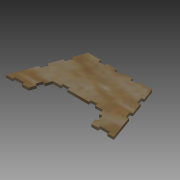
# Autodesk Inventor part: back
Saved by Autodesk Inventor 2016 (Build 200138000, 138)
## iProperties
Created: 2015-10-06
Part Number: back
Material: Generic
Document SubType Name: Modeling
Designer: Haukur
Density: 1 g/cm^3
Appearance: Plywood - Weathered
Author: Haukur
Autodesk Inventor part; units mm, degrees
ref_plane "YZ Plane" through (0, 0, 0) normal (1, 0, 0) x (0, 1, 0)
ref_plane "XZ Plane" through (0, 0, 0) normal (0, 1, 0) x (-1, 0, 0)
ref_plane "XY Plane" through (0, 0, 0) normal (0, 0, 1) x (1, 0, 0)
sketch "Sketch1" plane through (0, 0, 0) normal (0, 0, 1) x (1, 0, 0)
  line L0 (-6.8404, -18.7939) -> (73.1596, -18.7939) construction
  line L1 (126.5636, -18.7939) -> (116.303, 9.3969)
  line L2 (27.3616, 75.1754) -> (20.5212, 56.3816)
  line L3 (20.5212, 56.3816) -> (24.28, 55.0135)
  line L4 (24.28, 55.0135) -> (20.8598, 45.6166)
  line L5 (20.8598, 45.6166) -> (17.101, 46.9846)
  line L6 (17.101, 46.9846) -> (10.2606, 28.1908)
  line L7 (10.2606, 28.1908) -> (14.0194, 26.8227)
  line L8 (14.0194, 26.8227) -> (10.5992, 17.4258)
  line L9 (10.5992, 17.4258) -> (6.8404, 18.7939)
  line L10 (6.8404, 18.7939) -> (-6.8404, -18.7939)
  line L11 (27.3616, 75.1754) -> (47.3616, 75.1754)
  line L12 (47.3616, 75.1754) -> (47.3616, 71.1754)
  line L13 (47.3616, 71.1754) -> (57.3616, 71.1754)
  line L14 (57.3616, 71.1754) -> (57.3616, 75.1754)
  line L15 (57.3616, 75.1754) -> (72.3616, 75.1754)
  line L16 (72.3616, 75.1754) -> (72.3616, 71.1754)
  line L17 (72.3616, 71.1754) -> (82.3616, 71.1754)
  line L18 (82.3616, 71.1754) -> (82.3616, 75.1754)
  line L19 (82.3616, 75.1754) -> (97.3616, 75.1754)
  line L20 (97.3616, 75.1754) -> (97.3616, 71.1754)
  line L21 (97.3616, 71.1754) -> (107.3616, 71.1754)
  line L22 (107.3616, 71.1754) -> (107.3616, 75.1754)
  line L23 (107.3616, 75.1754) -> (127.3616, 75.1754)
  line L24 (-6.8404, -18.7939) -> (3.1596, -18.7939)
  line L25 (3.1596, -18.7939) -> (3.1596, -14.7939)
  line L26 (3.1596, -14.7939) -> (18.1596, -14.7939)
  line L27 (18.1596, -14.7939) -> (18.1596, -18.7939)
  line L28 (28.1596, -18.7939) -> (18.1596, -18.7939)
  line L29 (38.4202, 9.3969) -> (35, 0)
  line L30 (35, 0) -> (31.2412, 1.3681)
  line L31 (31.2412, 1.3681) -> (27.821, -8.0288)
  line L32 (27.821, -8.0288) -> (31.5798, -9.3969)
  line L33 (31.5798, -9.3969) -> (28.1596, -18.7939)
  line L34 (38.4202, 9.3969) -> (50.5212, 9.3969)
  line L35 (50.5212, 9.3969) -> (50.5212, 13.3969)
  line L36 (50.5212, 13.3969) -> (60.5212, 13.3969)
  line L37 (60.5212, 13.3969) -> (60.5212, 9.3969)
  line L38 (116.303, 9.3969) -> (104.202, 9.3969)
  line L39 (104.202, 9.3969) -> (104.202, 13.3969)
  line L40 (104.202, 13.3969) -> (94.202, 13.3969)
  line L41 (94.202, 13.3969) -> (94.202, 9.3969)
  line L42 (60.5212, 9.3969) -> (94.202, 9.3969)
  line L43 (116.303, 9.3969) -> (119.7232, 0)
  line L44 (119.7232, 0) -> (123.482, 1.3681)
  line L45 (123.482, 1.3681) -> (126.9022, -8.0288)
  line L46 (126.9022, -8.0288) -> (123.1434, -9.3969)
  line L47 (123.1434, -9.3969) -> (126.5636, -18.7939)
  line L48 (126.5636, -18.7939) -> (136.5636, -18.7939)
  line L49 (136.5636, -18.7939) -> (136.5636, -14.7939)
  line L50 (136.5636, -14.7939) -> (151.5636, -14.7939)
  line L51 (151.5636, -14.7939) -> (151.5636, -18.7939)
  line L52 (161.5636, -18.7939) -> (151.5636, -18.7939)
  line L53 (127.3616, 75.1754) -> (134.202, 56.3816)
  line L54 (134.202, 56.3816) -> (130.4432, 55.0135)
  line L55 (130.4432, 55.0135) -> (133.8634, 45.6166)
  line L56 (133.8634, 45.6166) -> (137.6222, 46.9846)
  line L57 (137.6222, 46.9846) -> (144.4626, 28.1908)
  line L58 (144.4626, 28.1908) -> (140.7038, 26.8227)
  line L59 (140.7038, 26.8227) -> (144.124, 17.4258)
  line L60 (144.124, 17.4258) -> (147.8828, 18.7939)
  line L61 (147.8828, 18.7939) -> (161.5636, -18.7939)
  dimension "d22" = 100
  dimension "d24" = 100
  dimension "d27" = 35
  dimension "d28" = 30
  dimension "d29" = 35
  dimension "d30" = 30
  dimension "d32" = 20
  dimension "d33" = 4
  dimension "d34" = 10
  dimension "d35" = 20
  dimension "d36" = 10
  dimension "d37" = 20
  dimension "d38" = 4
  dimension "d39" = 10
  dimension "d40" = 15
  dimension "d41" = 10
  dimension "d42" = 15
  dimension "d43" = 10
  dimension "d49" = 10
  dimension "d50" = 4
  dimension "d51" = 15
  dimension "d52" = 10
  dimension "d53" = 4
  dimension "d54" = 10
  dimension "d55" = 12.101
  dimension "d56" = 4
  dimension "d57" = 10
  dimension "d58" = 12.101
  dimension "d59" = 10
  dimension "d60" = 10
  dimension "d62" = 10
  dimension "d63" = 10
  dimension "d64" = 4
  dimension "d65" = 15
  dimension "d68" = 20
  dimension "d69" = 4
  dimension "d70" = 10
  dimension "d71" = 20
  dimension "d72" = 4
  dimension "d73" = 10
  constraints: 124 end point, 22 perpendicular, 9 point on line, 1 collinear, 1 horizontal
  measures "d22" distance of L0.start L2.start
  measures "d24" distance of L2.start L23.end
  measures "d27" distance of L52.start L1.start
  measures "d28" distance of L1.start L1.end
  measures "d29" distance of L0.start L28.start
  measures "d30" distance of L28.start L29.start
  measures "d32" distance of L2.start L2.end
  measures "d33" distance of L2.end L3.end
  measures "d34" distance of L3.end L4.end
  measures "d35" distance of L5.end L6.end
  measures "d36" distance of L7.end L8.end
  measures "d37" distance of L2.start L11.end
  measures "d38" distance of L11.end L12.end
  measures "d39" distance of L12.end L13.end
  measures "d40" distance of L14.end L15.end
  measures "d41" distance of L16.end L17.end
  measures "d42" distance of L18.end L19.end
  measures "d43" distance of L20.end L21.end
  measures "d49" distance of L0.start L24.end
  measures "d50" distance of L24.end L25.end
  measures "d51" distance of L25.end L26.end
  measures "d52" distance of L29.start L29.end
  measures "d53" distance of L29.end L30.end
  measures "d54" distance of L30.end L31.end
  measures "d55" distance of L29.start L34.end
  measures "d56" distance of L34.end L35.end
  measures "d57" distance of L35.end L36.end
  measures "d58" distance of L1.end L38.end
  measures "d59" distance of L39.end L40.end
  measures "d60" distance of L1.end L43.end
  measures "d62" distance of L44.end L45.end
  measures "d63" distance of L1.start L48.end
  measures "d64" distance of L48.end L49.end
  measures "d65" distance of L49.end L50.end
  measures "d68" distance of L23.end L53.end
  measures "d69" distance of L53.end L54.end
  measures "d70" distance of L54.end L55.end
  measures "d71" distance of L56.end L57.end
  measures "d72" distance of L57.end L58.end
  measures "d73" distance of L58.end L59.end
extrude "Extrusion1" add sketch "Sketch1" along normal blind 4 contours L1 L46 L45 L44 L38 L39 L40 L41 L42 L37 L36 L35 L34 L29 L30 L31 L32 L33 L28 L27 L26 L25 L24 L10 L9 L8 L7 L6 L5 L4 L3 L2 L11 L12 L13 L14 L15 L16 L17 L18 L19 L20 L21 L22 L23 L53 L54 L55 L56 L57 L58 L59 L60 L61 L52 L51 L50 L49 L48
body "Solid1"
